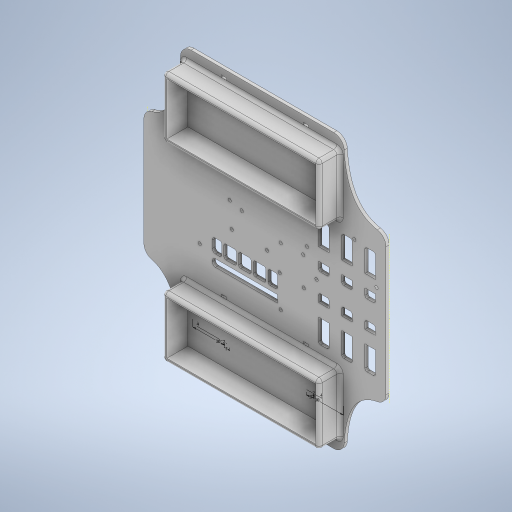
# Autodesk Inventor part: Part_base_plate
Saved by Autodesk Inventor 2023 (Build 270158000, 158)
## iProperties
Created: 2023-02-25
Part Number: Part_base_plate
Material: Generic
Document SubType Name: Modeling
Designer: geoff
Density: 1 g/cm^3
Appearance: Default
Author: geoff
Autodesk Inventor part; units mm, degrees
ref_plane "YZ Plane" through (0, 0, 0) normal (1, 0, 0) x (0, 1, 0)
ref_plane "XZ Plane" through (0, 0, 0) normal (0, 1, 0) x (-1, 0, 0)
ref_plane "XY Plane" through (0, 0, 0) normal (0, 0, 1) x (1, 0, 0)
sketch "Sketch1" plane through (0, 0, 0) normal (0, 0, 1) x (1, 0, 0)
  line L0 (0, 0) -> (186, 0)
  line L1 (186, 0) -> (186, 260)
  line L2 (186, 260) -> (0, 260)
  line L3 (0, 260) -> (-44, 260)
  line L4 (-44, 260) -> (-44, 0)
  line L5 (-44, 0) -> (0, 0)
  dimension "d1" = 260
  dimension "d121" = 230
  constraints: 12 end point, 2 horizontal, 2 parallel, 2 perpendicular
  measures "d1" distance of L0.end L1.end
  measures "d121" distance between parallel lines of L1 L4
extrude "Extrusion1" add sketch "Sketch1" along normal blind 3
sketch "Sketch2" plane through (0, 0, 3) normal (0, 0, 1) x (1, 0, 0)
  line L0 (186, 0) -> (186, 260) projected
  line L1 (186, 260) -> (146, 260)
  line L2 (186, 200) -> (186, 260)
  line L3 (0, 0) -> (186, 0) projected
  line L4 (186, 0) -> (146, 0)
  line L5 (186, 60) -> (186, 0)
  line L6 (146, 260) -> (146, 200) construction
  line L7 (146, 200) -> (186, 200) construction
  spline S0 degree 2 poles (146, 260) (146, 200) (186, 200) knots 1 1 1 2 2 2
  line L8 (186, 60) -> (146, 60) construction
  line L9 (146, 60) -> (146, 0) construction
  spline S1 degree 2 poles (186, 60) (146, 60) (146, 0) knots 1 1 1 2 2 2
  dimension "d4" = 40
  constraints: 8 end point, 2 horizontal, 6 other
  measures "d4" distance of L0.end L1.end
sketch "Sketch3" plane through (0, 0, 3) normal (0, 0, 1) x (1, 0, 0)
  line L0 (166, 101) -> (176, 101)
  line L1 (176, 101) -> (176, 79)
  line L2 (176, 79) -> (166, 79)
  line L3 (166, 79) -> (166, 101)
  line L4 (144, 101) -> (154, 101)
  line L5 (154, 101) -> (154, 79)
  line L6 (154, 79) -> (144, 79)
  line L7 (144, 79) -> (144, 101)
  line L8 (122, 101) -> (132, 101)
  line L9 (132, 101) -> (132, 79)
  line L10 (132, 79) -> (122, 79)
  line L11 (122, 79) -> (122, 101)
  line L12 (122, 181) -> (132, 181)
  line L13 (132, 181) -> (132, 159)
  line L14 (132, 159) -> (122, 159)
  line L15 (122, 159) -> (122, 181)
  line L16 (144, 181) -> (154, 181)
  line L17 (154, 181) -> (154, 159)
  line L18 (154, 159) -> (144, 159)
  line L19 (144, 159) -> (144, 181)
  line L20 (166, 181) -> (176, 181)
  line L21 (176, 181) -> (176, 159)
  line L22 (176, 159) -> (166, 159)
  line L23 (166, 159) -> (166, 181)
  line L24 (122, 147) -> (132, 147)
  line L25 (132, 147) -> (132, 139)
  line L26 (132, 139) -> (122, 139)
  line L27 (122, 139) -> (122, 147)
  line L28 (122, 121) -> (132, 121)
  line L29 (132, 121) -> (132, 113)
  line L30 (132, 113) -> (122, 113)
  line L31 (122, 113) -> (122, 121)
  line L32 (144, 147) -> (154, 147)
  line L33 (154, 147) -> (154, 139)
  line L34 (154, 139) -> (144, 139)
  line L35 (144, 139) -> (144, 147)
  line L36 (144, 121) -> (154, 121)
  line L37 (154, 121) -> (154, 113)
  line L38 (154, 113) -> (144, 113)
  line L39 (144, 113) -> (144, 121)
  line L40 (166, 147) -> (176, 147)
  line L41 (176, 147) -> (176, 139)
  line L42 (176, 139) -> (166, 139)
  line L43 (166, 139) -> (166, 147)
  line L44 (166, 121) -> (176, 121)
  line L45 (176, 121) -> (176, 113)
  line L46 (176, 113) -> (166, 113)
  line L47 (166, 113) -> (166, 121)
  line L48 (186, 0) -> (186, 260) projected
  line L49 (186, 200) -> (146, 200) projected
  line L50 (146, 60) -> (186, 60) projected
  line L51 (21, 100) -> (83, 100)
  line L52 (83, 100) -> (83, 93)
  line L53 (83, 93) -> (21, 93)
  line L54 (21, 93) -> (21, 100)
  line L55 (21, 117) -> (30, 117)
  line L56 (30, 117) -> (30, 104)
  line L57 (30, 104) -> (21, 104)
  line L58 (21, 104) -> (21, 117)
  line L59 (32, 117) -> (44, 117)
  line L60 (44, 117) -> (44, 104)
  line L61 (44, 104) -> (32, 104)
  line L62 (32, 104) -> (32, 117)
  line L63 (46, 117) -> (58, 117)
  line L64 (58, 117) -> (58, 104)
  line L65 (58, 104) -> (46, 104)
  line L66 (46, 104) -> (46, 117)
  line L67 (60, 117) -> (72, 117)
  line L68 (72, 117) -> (72, 104)
  line L69 (72, 104) -> (60, 104)
  line L70 (60, 104) -> (60, 117)
  line L71 (74, 117) -> (83, 117)
  line L72 (83, 117) -> (83, 104)
  line L73 (83, 104) -> (74, 104)
  line L74 (74, 104) -> (74, 117)
  line L75 (0, 0) -> (186, 0) projected
  line L76 (0, 260) -> (0, 0) projected
  point P0 (146, 0)
  dimension "d9" = 10
  dimension "d10" = 10
  dimension "d11" = 10
  dimension "d12" = 10
  dimension "d13" = 10
  dimension "d14" = 10
  dimension "d15" = 10
  dimension "d16" = 10
  dimension "d17" = 12
  dimension "d18" = 10
  dimension "d19" = 12
  dimension "d20" = 10
  dimension "d21" = 22
  dimension "d22" = 22
  dimension "d23" = 8
  dimension "d24" = 8
  dimension "d25" = 8
  dimension "d26" = 8
  dimension "d27" = 19
  dimension "d28" = 19
  dimension "d29" = 12
  dimension "d30" = 12
  dimension "d31" = 93
  dimension "d32" = 7
  dimension "d33" = 21
  dimension "d34" = 4
  dimension "d35" = 9
  dimension "d36" = 2
  dimension "d37" = 12
  dimension "d38" = 2
  dimension "d39" = 12
  dimension "d40" = 2
  dimension "d41" = 12
  dimension "d42" = 62
  dimension "d43" = 13
  dimension "d44" = 4
  dimension "d45" = 0
  dimension "d46" = 9
  dimension "d47" = 2
  dimension "d48" = 39
  dimension "d49" = 13
  constraints: 144 end point, 38 point on line, 36 parallel, 18 horizontal, 18 perpendicular
  measures "d9" distance between parallel lines of L48 L21
  measures "d10" distance between parallel lines of L48 L1
  measures "d11" distance between parallel lines of L48 L41
  measures "d12" distance between parallel lines of L48 L45
  measures "d13" distance of L21.end L22.end
  measures "d14" distance of L41.end L42.end
  measures "d15" distance of L45.end L46.end
  measures "d16" distance of L0.start L0.end
  measures "d17" distance between parallel lines of L23 L17
  measures "d18" distance of L17.end L18.end
  measures "d19" distance between parallel lines of L19 L13
  measures "d20" distance of L13.end L14.end
  measures "d21" distance of L14.end L12.start
  measures "d22" distance of L10.end L8.start
  measures "d23" distance of L30.end L28.start
  measures "d24" distance of L38.end L36.start
  measures "d25" distance of L46.end L44.start
  measures "d26" distance of L26.end L24.start
  measures "d27" distance between parallel lines of L49 L20
  measures "d28" distance between parallel lines of L50 L2
  measures "d29" distance between parallel lines of L24 L14
  measures "d30" distance between parallel lines of L30 L8
  measures "d31" distance between parallel lines of L75 L53
  measures "d32" distance of L53.end L51.start
  measures "d33" distance between parallel lines of L76 L54
  measures "d34" distance between parallel lines of L51 L57
  measures "d35" distance of L56.end L57.end
  measures "d36" distance between parallel lines of L62 L56
  measures "d37" distance of L60.end L61.end
  measures "d38" distance between parallel lines of L66 L60
  measures "d39" distance of L64.end L65.end
  measures "d40" distance between parallel lines of L70 L64
  measures "d41" distance of L68.end L69.end
  measures "d42" distance of L52.end L53.end
  measures "d43" distance of L71.end L72.end
  measures "d44" distance between parallel lines of L51 L73
  measures "d45" distance between parallel lines of L52 L72
  measures "d46" distance of L72.end L73.end
  measures "d47" distance between parallel lines of L68 L74
  measures "d48" distance between parallel lines of L11 L52
  measures "d49" distance of L57.end L55.start
extrude "Extrusion3" cut sketch "Sketch3" against normal blind 5
sketch "Sketch4" plane through (0, 0, 3) normal (0, 0, 1) x (1, 0, 0)
  circle A0 centre (177, 153) radius 1.5
  line L0 (186, 0) -> (186, 260) projected
  line L1 (186, 200) -> (146, 200) projected
  circle A1 centre (107.5, 145) radius 1.5
  circle A2 centre (120, 131) radius 1.5
  circle A3 centre (111, 153.5) radius 1.5
  circle A4 centre (156, 182) radius 1.5
  circle A5 centre (108, 118) radius 1.5
  circle A6 centre (85, 119) radius 1.5
  circle A7 centre (86, 144) radius 1.5
  circle A8 centre (73, 131.5) radius 1.5
  circle A9 centre (86, 89) radius 1.5
  line L2 (146, 60) -> (186, 60) projected
  circle A10 centre (9, 105) radius 1.5
  line L3 (0, 260) -> (0, 0) projected
  line L4 (0, 0) -> (186, 0) projected
  circle A11 centre (39.5, 132) radius 1.5
  circle A12 centre (37.5, 155) radius 1.5
  circle A13 centre (49, 152) radius 1.5
  point P0 (146, 0)
  dimension "d124" = 35
  dimension "d52" = 9
  dimension "d53" = 47
  dimension "d54" = 3
  dimension "d55" = 55
  dimension "d56" = 78.5
  dimension "d57" = 3
  dimension "d58" = 3
  dimension "d59" = 66
  dimension "d60" = 69
  dimension "d61" = 46.5
  dimension "d62" = 75
  dimension "d63" = 3
  dimension "d64" = 18
  dimension "d65" = 30
  dimension "d66" = 3
  dimension "d67" = 78
  dimension "d68" = 3
  dimension "d69" = 82
  dimension "d70" = 101
  dimension "d71" = 3
  dimension "d73" = 81
  dimension "d74" = 100
  dimension "d75" = 56
  dimension "d76" = 3
  dimension "d77" = 3
  dimension "d78" = 68.5
  dimension "d79" = 113
  dimension "d80" = 3
  dimension "d81" = 100
  dimension "d82" = 29
  dimension "d83" = 3
  dimension "d84" = 9
  dimension "d85" = 105
  dimension "d86" = 3
  dimension "d87" = 68
  dimension "d88" = 39.5
  dimension "d89" = 3
  dimension "d90" = 45
  dimension "d91" = 37.5
  dimension "d92" = 3
  dimension "d93" = 49
  dimension "d94" = 48
  constraints: 14 centre point
  measures "d52" distance from line of L0 A0.centre
  measures "d53" distance from line of A0.centre L1
  measures "d54" diameter of A0
  measures "d55" distance from line of L1 A1.centre
  measures "d56" distance from line of L0 A1.centre
  measures "d57" diameter of A1
  measures "d58" diameter of A2
  measures "d59" distance from line of L0 A2.centre
  measures "d60" distance from line of L1 A2.centre
  measures "d61" distance from line of L1 A3.centre
  measures "d62" distance from line of L0 A3.centre
  measures "d63" diameter of A3
  measures "d64" distance from line of L1 A4.centre
  measures "d65" distance from line of L0 A4.centre
  measures "d66" diameter of A4
  measures "d67" distance from line of L0 A5.centre
  measures "d68" diameter of A5
  measures "d69" distance from line of A5.centre L1
  measures "d70" distance from line of L0 A6.centre
  measures "d71" diameter of A6
  measures "d73" distance from line of A6.centre L1
  measures "d74" distance from line of L0 A7.centre
  measures "d75" distance from line of A7.centre L1
  measures "d76" diameter of A7
  measures "d77" diameter of A8
  measures "d78" distance from line of L1 A8.centre
  measures "d79" distance from line of L0 A8.centre
  measures "d80" diameter of A9
  measures "d81" distance from line of L0 A9.centre
  measures "d82" distance from line of L2 A9.centre
  measures "d83" diameter of A10
  measures "d84" distance from line of L3 A10.centre
  measures "d85" distance from line of L4 A10.centre
  measures "d86" diameter of A11
  measures "d87" distance from line of L1 A11.centre
  measures "d88" distance from line of L3 A11.centre
  measures "d89" diameter of A12
  measures "d90" distance from line of L1 A12.centre
  measures "d91" distance from line of L3 A12.centre
  measures "d92" diameter of A13
  measures "d93" distance from line of L3 A13.centre
  measures "d94" distance from line of L1 A13.centre
sketch "Sketch5" plane through (0, 0, 3) normal (0, 0, 1) x (1, 0, 0)
  circle A0 centre (76, 181) radius 1.3334
  line L0 (186, 200) -> (146, 200) projected
  line L1 (0, 260) -> (0, 0) projected
  dimension "d95" = 19
  dimension "d96" = 76
  constraints: 1 centre point
  measures "d95" distance from line of L0 A0.centre
  measures "d96" distance from line of L1 A0.centre
extrude "Extrusion4" cut sketch "Sketch4" against normal blind 5
extrude "Extrusion5" cut sketch "Sketch5" against normal blind 5
fillet "Fillet1" radius 2 24 edges at (176, 181, 1.5) (154, 181, 1.5) (166, 181, 1.5) (144, 181, 1.5) (122, 181, 1.5) (132, 181, 1.5) (132, 121, 1.5) (154, 121, 1.5) (122, 121, 1.5) (144, 121, 1.5) (166, 121, 1.5) (176, 121, 1.5) (166, 139, 1.5) (144, 139, 1.5) (122, 139, 1.5) (132, 139, 1.5) (154, 139, 1.5) (176, 139, 1.5) (176, 79, 1.5) (154, 79, 1.5) (166, 79, 1.5) (144, 79, 1.5) (122, 79, 1.5) (132, 79, 1.5)
sketch "Sketch8" plane through (0, 0, 0) normal (0, 0, -1) x (-1, 0, 0)
  line L0 (44, 260) -> (9, 260)
  line L1 (-186, 260) -> (44, 260) construction
  line L2 (44, 260) -> (44, 190)
  line L3 (9, 260) -> (9, 190) construction
  line L4 (9, 190) -> (44, 190) construction
  spline S0 degree 2 poles (9, 260) (9, 190) (44, 190) knots 1 1 1 2 2 2
  line L5 (44, 0) -> (-186, 0) construction
  line L6 (44, 0) -> (44, 70)
  line L7 (44, 0) -> (9, 0)
  line L8 (44, 0) -> (-186, 0) projected
  line L9 (44, 70) -> (9, 70) construction
  line L10 (9, 70) -> (9, 0) construction
  spline S1 degree 2 poles (44, 70) (9, 70) (9, 0) knots 1 1 1 2 2 2
  point P0 (0, 0)
  point P1 (-146, 260)
  point P2 (-146, 0)
  dimension "d124" = 35
  dimension "d125" = 70
  dimension "d126" = 70
  dimension "d127" = 35
  constraints: 8 end point, 2 horizontal, 2 point on line, 2 vertical, 6 other
  measures "d124" distance of L0.start L0.end
  measures "d125" distance of L0.start L2.end
  measures "d126" distance of L5.start L6.end
  measures "d127" distance of L5.start L7.end
extrude "Extrusion7" cut sketch "Sketch8" against normal blind 10
extrude "Extrusion8" cut sketch "Sketch2" against normal blind 10
fillet "Fillet2" radius 3 4 edges at (21, 117, 1.5) (21, 104, 1.5) (21, 93, 1.5) (21, 100, 1.5)
fillet "Fillet3" radius 2 18 edges at (32, 104, 1.5) (46, 104, 1.5) (60, 104, 1.5) (74, 104, 1.5) (74, 117, 1.5) (60, 117, 1.5) (46, 117, 1.5) (32, 117, 1.5) (83, 117, 1.5) (72, 117, 1.5) (58, 117, 1.5) (44, 117, 1.5) (30, 117, 1.5) (83, 104, 1.5) (72, 104, 1.5) (58, 104, 1.5) (44, 104, 1.5) (30, 104, 1.5)
sketch "Sketch9" plane through (0, 0, 0) normal (0, 0, -1) x (-1, 0, 0)
  line L0 (-29.5, 32.6739) -> (-34.5, 32.6739)
  line L1 (-34.5, 32.6739) -> (-34.5, 30.6739)
  line L2 (-34.5, 30.6739) -> (-29.5, 30.6739)
  line L3 (-29.5, 30.6739) -> (-29.5, 32.6739)
  line L4 (-142.5, 36.6739) -> (0.5, 36.6739) projected
  line L5 (0.5, 36.6739) -> (0.5, 67.6739) projected
  line L6 (-107.5, 32.6739) -> (-112.5, 32.6739)
  line L7 (-112.5, 32.6739) -> (-112.5, 30.6739)
  line L8 (-112.5, 30.6739) -> (-107.5, 30.6739)
  line L9 (-107.5, 30.6739) -> (-107.5, 32.6739)
  line L10 (-142.5, 67.6739) -> (-142.5, 36.6739) projected
  line L11 (-139.5, 64.6739) -> (-139.5, 39.6739) construction
  line L12 (-139.5, 52.1739) -> (-2.5, 52.1739) construction
  line L13 (-2.5, 39.6739) -> (-2.5, 64.6739) construction
  line L14 (-29.5, 71.6739) -> (-34.5, 71.6739)
  line L15 (-34.5, 71.6739) -> (-34.5, 73.6739)
  line L16 (-34.5, 73.6739) -> (-29.5, 73.6739)
  line L17 (-29.5, 73.6739) -> (-29.5, 71.6739)
  line L18 (-107.5, 71.6739) -> (-112.5, 71.6739)
  line L19 (-112.5, 71.6739) -> (-112.5, 73.6739)
  line L20 (-112.5, 73.6739) -> (-107.5, 73.6739)
  line L21 (-107.5, 73.6739) -> (-107.5, 71.6739)
  line L22 (-186, 60) -> (-186, 200) construction
  line L23 (-186, 130) -> (44, 130) construction
  line L24 (44, 190) -> (44, 70) construction
  line L25 (-29.5, 227.3261) -> (-34.5, 227.3261)
  line L26 (-34.5, 227.3261) -> (-34.5, 229.3261)
  line L27 (-34.5, 229.3261) -> (-29.5, 229.3261)
  line L28 (-29.5, 229.3261) -> (-29.5, 227.3261)
  line L29 (-107.5, 227.3261) -> (-112.5, 227.3261)
  line L30 (-112.5, 227.3261) -> (-112.5, 229.3261)
  line L31 (-112.5, 229.3261) -> (-107.5, 229.3261)
  line L32 (-107.5, 229.3261) -> (-107.5, 227.3261)
  line L33 (-34.5, 186.3261) -> (-29.5, 186.3261)
  line L34 (-34.5, 188.3261) -> (-34.5, 186.3261)
  line L35 (-29.5, 188.3261) -> (-34.5, 188.3261)
  line L36 (-29.5, 186.3261) -> (-29.5, 188.3261)
  line L37 (-112.5, 186.3261) -> (-107.5, 186.3261)
  line L38 (-112.5, 188.3261) -> (-112.5, 186.3261)
  line L39 (-107.5, 188.3261) -> (-112.5, 188.3261)
  line L40 (-107.5, 186.3261) -> (-107.5, 188.3261)
  point P0 (0, 0)
  point P1 (-32, 32.6739)
  point P2 (-32, 227.3261)
  dimension "d134" = 5
  dimension "d135" = 2
  dimension "d136" = 4
  dimension "d137" = 30
  dimension "d138" = 5
  dimension "d139" = 2
  dimension "d140" = 4
  dimension "d141" = 30
  constraints: 68 end point, 25 symmetric about line, 5 midpoint, 4 parallel, 2 horizontal, 2 perpendicular
  measures "d134" distance of L1.end L2.end
  measures "d135" distance of L2.end L0.start
  measures "d136" distance from line of L4 point (-32, 32.674)
  measures "d137" distance between parallel lines of L3 L5
  measures "d138" distance of L7.end L8.end
  measures "d139" distance of L6.end L7.end
  measures "d140" distance between parallel lines of L4 L6
  measures "d141" distance between parallel lines of L7 L10
sketch "Sketch10" plane through (0, 0, 3) normal (0, 0, 1) x (1, 0, 0)
  line L0 (-2.2, 15) -> (139.2, 15)
  line L1 (139.2, 15) -> (139.2, 64.6)
  line L2 (139.2, 64.6) -> (-2.2, 64.6)
  line L3 (-2.2, 64.6) -> (-2.2, 15)
  line L4 (-9, 0) -> (146, 0) projected
  line L5 (-6.2, 11) -> (142.3138, 11)
  line L6 (142.3138, 11) -> (142.3138, 68.6)
  line L7 (142.3138, 68.6) -> (-6.2, 68.6)
  line L8 (-6.2, 68.6) -> (-6.2, 11)
  line L9 (-44, 190) -> (-44, 70) construction
  line L10 (-44, 130) -> (186, 130) construction
  line L11 (186, 60) -> (186, 200) construction
  line L12 (-2.2, 245) -> (139.2, 245)
  line L13 (139.2, 245) -> (139.2, 195.4)
  line L14 (139.2, 195.4) -> (-2.2, 195.4)
  line L15 (-2.2, 195.4) -> (-2.2, 245)
  line L16 (-6.2, 249) -> (142.3138, 249)
  line L17 (142.3138, 249) -> (142.3138, 191.4)
  line L18 (142.3138, 191.4) -> (-6.2, 191.4)
  line L19 (-6.2, 191.4) -> (-6.2, 249)
  point P0 (0, 0)
  dimension "d146" = 141.4
  dimension "d147" = 49.6
  dimension "d148" = 15
  dimension "d149" = 6.8
  dimension "d150" = 4
  dimension "d151" = 4
  dimension "d152" = 4
  dimension "d153" = 3.1138
  constraints: 34 end point, 8 symmetric about line, 4 parallel, 2 horizontal, 2 midpoint, 2 perpendicular
  measures "d146" distance of L1.end L2.end
  measures "d147" distance of L2.end L0.start
  measures "d148" distance between parallel lines of L4 L0
  measures "d149" horizontal distance of L4.start L0.start
  measures "d150" distance between parallel lines of L2 L7
  measures "d151" distance between parallel lines of L8 L3
  measures "d152" distance between parallel lines of L5 L0
  measures "d153" distance between parallel lines of L1 L6
extrude "Extrusion11" add sketch "Sketch10" along normal blind 20
sketch "Sketch11" plane through (0, 0, 3) normal (0, 0, 1) x (1, 0, 0)
  line L0 (-2.2, 64.6) -> (-2.2, 15) construction
  line L1 (-2.2, 39.8) -> (139.2, 39.8) construction
  line L2 (139.2, 15) -> (139.2, 64.6) construction
  line L3 (139.2, 195.4) -> (139.2, 245) construction
  line L4 (139.2, 220.2) -> (-2.2, 220.2) construction
  line L5 (-2.2, 245) -> (-2.2, 195.4) construction
  line L6 (29.5, 73.6739) -> (34.5, 73.6739) projected
  line L7 (34.5, 73.6739) -> (34.5, 71.6739) projected
  line L8 (34.5, 71.6739) -> (29.5, 71.6739) projected
  line L9 (29.5, 71.6739) -> (29.5, 73.6739) projected
  line L10 (112.5, 71.6739) -> (107.5, 71.6739) projected
  line L11 (107.5, 71.6739) -> (107.5, 73.6739) projected
  line L12 (107.5, 73.6739) -> (112.5, 73.6739) projected
  line L13 (112.5, 73.6739) -> (112.5, 71.6739) projected
  line L14 (107.5, 186.3261) -> (107.5, 188.3261) projected
  line L15 (107.5, 188.3261) -> (112.5, 188.3261) projected
  line L16 (112.5, 188.3261) -> (112.5, 186.3261) projected
  line L17 (112.5, 186.3261) -> (107.5, 186.3261) projected
  line L18 (29.5, 186.3261) -> (29.5, 188.3261) projected
  line L19 (29.5, 188.3261) -> (34.5, 188.3261) projected
  line L20 (34.5, 186.3261) -> (29.5, 186.3261) projected
  line L21 (34.5, 188.3261) -> (34.5, 186.3261) projected
  line L22 (29.5, 5.9261) -> (34.5, 5.9261)
  line L23 (34.5, 5.9261) -> (34.5, 7.9261)
  line L24 (34.5, 7.9261) -> (29.5, 7.9261)
  line L25 (29.5, 7.9261) -> (29.5, 5.9261)
  line L26 (112.5, 7.9261) -> (107.5, 7.9261)
  line L27 (107.5, 7.9261) -> (107.5, 5.9261)
  line L28 (107.5, 5.9261) -> (112.5, 5.9261)
  line L29 (112.5, 5.9261) -> (112.5, 7.9261)
  line L30 (107.5, 254.0739) -> (107.5, 252.0739)
  line L31 (107.5, 252.0739) -> (112.5, 252.0739)
  line L32 (112.5, 252.0739) -> (112.5, 254.0739)
  line L33 (112.5, 254.0739) -> (107.5, 254.0739)
  line L34 (29.5, 254.0739) -> (29.5, 252.0739)
  line L35 (29.5, 252.0739) -> (34.5, 252.0739)
  line L36 (34.5, 254.0739) -> (29.5, 254.0739)
  line L37 (34.5, 252.0739) -> (34.5, 254.0739)
  point P0 (0, 0)
  constraints: 36 end point, 16 symmetric about line, 4 midpoint
extrude "Extrusion12" cut sketch "Sketch11" against normal blind 20
fillet "Fillet4" radius 3 24 edges at (142.3138, 39.8, 3) (142.3138, 68.6, 13) (68.0569, 68.6, 3) (68.0569, 11, 3) (142.3138, 11, 13) (-6.2, 39.8, 3) (-6.2, 11, 13) (-6.2, 68.6, 13) (68.0569, 68.6, 23) (142.3138, 39.8, 23) (68.0569, 11, 23) (-6.2, 39.8, 23) (142.3138, 220.2, 3) (68.0569, 249, 3) (142.3138, 249, 13) (142.3138, 191.4, 13) (68.0569, 191.4, 3) (-6.2, 220.2, 3) (-6.2, 191.4, 13) (-6.2, 249, 13) (68.0569, 249, 23) (142.3138, 220.2, 23) (68.0569, 191.4, 23) (-6.2, 220.2, 23)
fillet "Fillet5" radius 10 8 edges at (-9, 260, 1.5) (-44, 190, 1.5) (146, 260, 1.5) (186, 200, 1.5) (186, 60, 1.5) (146, 0, 1.5) (-9, 0, 1.5) (-44, 70, 1.5)
body "Solid1"
